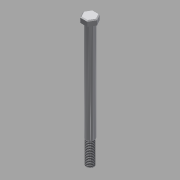
# Autodesk Inventor part: Axel
Saved by Autodesk Inventor 2013 (Build 170138000, 138)
## iProperties
Created: 2013-01-18
Part Number: Axel
Material: Aluminum 6061-AHC
Document SubType Name: Modeling
Designer: Naphat
Density: 1 g/cm^3
Author: Naphat
Autodesk Inventor part; units mm, degrees
ref_plane "YZ Plane" through (0, 0, 0) normal (1, 0, 0) x (0, 1, 0)
ref_plane "XZ Plane" through (0, 0, 0) normal (0, 1, 0) x (-1, 0, 0)
ref_plane "XY Plane" through (0, 0, 0) normal (0, 0, 1) x (1, 0, 0)
sketch "Sketch1" plane through (0, 0, 0) normal (0, 1, 0) x (-1, 0, 0)
  circle A0 centre (0, 0) radius 5
  dimension "d0" = 10
  constraints: 1 centre point, 1 coincident
  measures "d0" diameter of A0
extrude "Extrusion1" add sketch "Sketch1" along normal blind 140
sketch "Sketch2" plane through (0, 140, 0) normal (0, 1, 0) x (1, 0, 0)
  line L0 (4, -7) -> (-4, -7)
  line L1 (-4, -7) -> (-8.0005, -0.0709)
  line L2 (-4, -7) -> (4.001, -7) construction
  line L3 (-8.0005, -0.0709) -> (-4, 6.8581)
  line L4 (-4, 6.8581) -> (4.001, 6.8581)
  line L5 (4.001, 6.8581) -> (8.0015, -0.0709)
  line L6 (8.0015, -0.0709) -> (4, -7)
  dimension "d5" = 8
  dimension "d6" = 8.001
  dimension "d7" = 120
  dimension "d8" = 8.001
  dimension "d9" = 120
  dimension "d10" = 8.001
  dimension "d11" = 120
  dimension "d12" = 8.001
  dimension "d13" = 120
  constraints: 14 end point, 2 parallel, 1 equal length, 1 horizontal
  measures "d5" distance of L0.start L0.end
  measures "d6" distance of L0.end L1.end
  measures "d7" angle of L2 L1
  measures "d8" distance of L1.end L3.end
  measures "d9" angle of L1 L3
  measures "d10" distance of L3.end L4.end
  measures "d11" angle of L3 L4
  measures "d12" distance of L4.end L5.end
  measures "d13" angle of L4 L5
extrude "Extrusion2" add sketch "Sketch2" along normal blind 6
chamfer "Chamfer1" distance 1 angle 45 6 edges at (0, 146, 7) (-6.0002, 146, 3.5355) (6.0008, 146, 3.5355) (6.0013, 146, -3.3936) (0.0005, 146, -6.8581) (-6.0002, 146, -3.3936)
sketch "Sketch3" plane through (0, 0, 0) normal (0, -1, 0) x (1, 0, 0)
  circle A0 centre (0, 0) radius 5 projected
extrude "Extrusion3" cut sketch "Sketch3" against normal blind 26
sketch "Sketch4" plane through (0, 26, 0) normal (0, -1, 0) x (1, 0, 0)
  circle A0 centre (0, 0) radius 5 projected
  circle A1 centre (0, 0) radius 4.3197
  constraints: 1 centre point, 1 coincident
extrude "Extrusion4" add sketch "Sketch4" along normal blind 26 contours A1
fillet "Fillet1" radius 1 1 edges at (5, 26, 0)
thread "Thread1" size "3/8-16 UNC" class "2A" standard "ANSI Unified Screw Threads" full length
body "Solid1"
